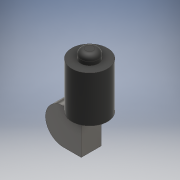
# Autodesk Inventor part: TS-40GZ7090
Saved by Autodesk Inventor 2017 SP1 (Build 210196100, 196)
## iProperties
Created: 2019-10-26
Part Number: TS-40GZ7090
Material: Stainless Steel
Document SubType Name: Modeling
Designer: Dell
Density: 8 g/cm^3
Appearance: Semi-Polished
Author: Dell
Autodesk Inventor part; units mm, degrees
ref_plane "YZ Plane" through (0, 0, 0) normal (1, 0, 0) x (0, 1, 0)
ref_plane "XZ Plane" through (0, 0, 0) normal (0, 1, 0) x (-1, 0, 0)
ref_plane "XY Plane" through (0, 0, 0) normal (0, 0, 1) x (1, 0, 0)
sketch "Sketch1" plane through (0, 0, 0) normal (0, 0, 1) x (1, 0, 0)
  circle A0 centre (0, 0) radius 35
  dimension "d0" = 70
  constraints: 1 centre point, 1 coincident
  measures "d0" diameter of A0
extrude "Extrusion1" add sketch "Sketch1" along normal blind 90
sketch "Sketch2" plane through (0, 0, 0) normal (0, 1, 0) x (-1, 0, 0)
  circle A0 centre (-35, -35) radius 35
  line L0 (35, 90) -> (-35, 90) projected
  line L1 (-35, 0) -> (35, 0) projected
  line L2 (0, 0) -> (0, -70)
  line L3 (0, -70) -> (-35, -70)
  line L4 (-35, 0) -> (35, 0) projected
  line L5 (-35, 0) -> (0, 0)
  dimension "d3" = 70
  constraints: 6 end point, 2 point on circle, 1 centre point, 1 horizontal, 1 perpendicular, 1 tangent, 1 vertical, 1 vertical alignment
  measures "d3" diameter of A0
extrude "Extrusion2" add sketch "Sketch2" along normal blind 37.5 and the other way blind 16.5
sketch "Sketch4" plane through (0, 37.5, 0) normal (0, 1, 0) x (1, 0, 0)
  arc A0 (35, 0) -> (35, 70) centre (35, 35) ccw projected
  circle A1 centre (10, 35) radius 3
  circle A2 centre (47.5, 13.3494) radius 3
  circle A3 centre (47.5, 56.6506) radius 3
  point P0 (0, 0)
  dimension "d8" = 25
  dimension "d9" = 6
  dimension "d12" = 360
  constraints: 3 centre point, 1 horizontal alignment, 7 other
  measures "d8" distance of A1.centre A0.centre
  measures "d9" diameter of A1
extrude "Extrusion3" cut sketch "Sketch4" against normal blind 15
sketch "Sketch5" plane through (0, 37.5, 0) normal (0, 1, 0) x (1, 0, 0)
  circle A0 centre (35, 35) radius 6
  arc A1 (35, 0) -> (35, 70) centre (35, 35) ccw projected
  point P0 (0, 0)
  dimension "d16" = 12
  constraints: 1 centre point, 1 coincident
  measures "d16" diameter of A0
extrude "Extrusion4" add sketch "Sketch5" along normal blind 14
sketch "Sketch6" plane through (35, 51.5, -35) normal (0, 1, 0) x (1, 0, 0)
  circle A0 centre (0, 0) radius 4
  arc A1 (0, -35) -> (0, 35) centre (0, 0) ccw projected
  point P0 (-35, -35)
  dimension "d19" = 8
  constraints: 1 centre point, 1 coincident
  measures "d19" diameter of A0
extrude "Extrusion5" add sketch "Sketch6" along normal blind 20
sketch "Sketch7" plane through (0, 0, 90) normal (0, 0, 1) x (1, 0, 0)
  circle A0 centre (0, 0) radius 17.5
  dimension "d22" = 35
  constraints: 1 centre point, 1 coincident
  measures "d22" diameter of A0
extrude "Extrusion6" add sketch "Sketch7" along normal blind 17
mirror "Mirror1" about plane through (0, 0, 0) normal (1, 0, 0) remove original yes
sketch "Sketch8" plane through (-35, 37.5, 0) normal (0, 1, 0) x (1, 0, 0)
  circle A0 centre (0, 35) radius 6 projected
  circle A1 centre (-12.5, 13.3494) radius 3 projected
  circle A2 centre (25, 35) radius 3 projected
  circle A3 centre (-12.5, 56.6506) radius 3 projected
  arc A4 (0, 70) -> (0, 0) centre (0, 35) ccw projected
  line L0 (35, 0) -> (0, 0) projected
  line L1 (35, 70) -> (35, 0) projected
  line L2 (0, 70) -> (35, 70) projected
  circle A5 centre (-12.5, 13.3494) radius 6.5
  circle A6 centre (-12.5, 56.6506) radius 6.5
  circle A7 centre (25, 35) radius 3 projected
  circle A8 centre (25, 35) radius 6.5
  dimension "d25" = 13
  dimension "d26" = 13
  dimension "d27" = 13
  constraints: 3 centre point, 3 coincident
  measures "d25" diameter of A5
  measures "d26" diameter of A6
  measures "d27" diameter of A8
extrude "Extrusion7" cut sketch "Sketch8" against normal blind 15 contours L2 L1 L0 A4
fillet "Fillet1" radius 10 1 edges at (17.5, 0, 107)
body "Solid1"
